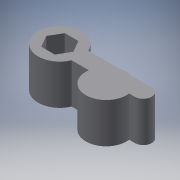
# Autodesk Inventor part: wingnut
Saved by Autodesk Inventor 2018 (Build 220112000, 112)
## iProperties
Created: 2018-11-24
Part Number: wingnut
Material: Generic
Document SubType Name: Modeling
Designer: Prakash
Density: 1 g/cm^3
Appearance: Default
Author: Prakash
Autodesk Inventor part; units mm, degrees
ref_plane "YZ Plane" through (0, 0, 0) normal (1, 0, 0) x (0, 1, 0)
ref_plane "XZ Plane" through (0, 0, 0) normal (0, 1, 0) x (-1, 0, 0)
ref_plane "XY Plane" through (0, 0, 0) normal (0, 0, 1) x (1, 0, 0)
sketch "Sketch1" plane through (0, 0, 0) normal (0, 0, 1) x (1, 0, 0)
  circle A0 centre (0, 0) radius 6.525
  line L0 (-2.0352, -3.525) -> (-4.0703, 0)
  line L1 (-4.0703, 0) -> (-2.0352, 3.525)
  line L2 (-2.0352, 3.525) -> (2.0352, 3.525)
  line L3 (2.0352, 3.525) -> (4.0703, 0)
  line L4 (4.0703, 0) -> (2.0352, -3.525)
  line L5 (2.0352, -3.525) -> (-2.0352, -3.525)
  line L6 (-4.0703, 0) -> (4.0703, 0) construction
  arc A1 (25, -2.5) -> (25, 2.5) centre (25, 0) ccw
  circle A2 centre (17.2205, -3.3329) radius 6.096
  line L7 (25, 2.5) -> (18.992, 2.5)
  line L8 (6.0271, 2.5) -> (15.449, 2.5)
  line L9 (6.0271, -2.5) -> (11.1817, -2.5)
  line L10 (23.2593, -2.5) -> (25, -2.5)
  dimension "d0" = 7.05
  dimension "d1" = 3
  dimension "d7" = 5
  dimension "d11" = 25
  dimension "d12" = 12.192
  dimension "d13" = 5.8329
  dimension "d14" = 7.7795
  constraints: 22 end point, 8 point on circle, 6 horizontal, 3 centre point, 2 coincident, 2 collinear, 2 tangent, 14 other
  measures "d0" distance between parallel lines of L2 L5
  measures "d1" distance edge to line of A0 L2
  measures "d7" distance between parallel lines of L9 L8
  measures "d11" distance of point (0, 0) A1.centre
  measures "d12" diameter of A2
  measures "d13" distance from line of L8 A2.centre
  measures "d14" horizontal distance of A1.centre A2.centre
extrude "Extrusion2" add sketch "Sketch1" along normal blind 12
body "Solid2"
